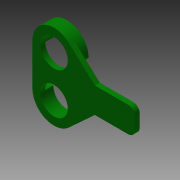
# Autodesk Inventor part: Down Sensor Holder
Saved by Autodesk Inventor 2014 (Build 180170000, 170)
## iProperties
Created: 2016-02-03
Part Number: Down Sensor Holder
Material: Generic
Document SubType Name: Modeling
Designer: Paul
Density: 1 g/cm^3
Appearance: Dark Green
Author: Paul
Autodesk Inventor part; units mm, degrees
ref_plane "YZ Plane" through (0, 0, 0) normal (1, 0, 0) x (0, 1, 0)
ref_plane "XZ Plane" through (0, 0, 0) normal (0, 1, 0) x (-1, 0, 0)
ref_plane "XY Plane" through (0, 0, 0) normal (0, 0, 1) x (1, 0, 0)
sketch "Sketch1" plane through (0, 0, 0) normal (0, 1, 0) x (-1, 0, 0)
  line L0 (-6, 8) -> (15, 8)
  line L1 (15, -8) -> (-6, -8)
  circle A0 centre (40.6, 13.025) radius 8.6
  circle A1 centre (40.6, -13.025) radius 8.6
  line L2 (15, 8) -> (31.4076, 23.048)
  line L3 (54.2, 13.025) -> (54.2, -13.025)
  line L4 (31.4076, -23.048) -> (15, -8)
  line L5 (-10, 0) -> (54.2, 0) construction
  line L6 (32, 21.625) -> (49.2, 21.625) construction
  line L7 (49.2, 21.625) -> (49.2, -21.625) construction
  line L8 (49.2, -21.625) -> (32, -21.625) construction
  line L9 (32, -21.625) -> (32, 21.625) construction
  line L10 (-10, 4) -> (-10, -4)
  arc A2 (-6, 8) -> (-10, 4) centre (-6, 4) ccw
  arc A3 (-10, -4) -> (-6, -8) centre (-6, -4) ccw
  arc A4 (31.4076, -23.048) -> (54.2, -13.025) centre (40.6, -13.025) ccw
  arc A5 (54.2, 13.025) -> (31.4076, 23.048) centre (40.6, 13.025) ccw
  arc A6 (31.4076, 23.048) -> (27, 13.025) centre (40.6, 13.025) ccw construction
  line L11 (32, 13.025) -> (27, 13.025) construction
  line L12 (32, -13.025) -> (27, -13.025) construction
  arc A7 (27, -13.025) -> (31.4076, -23.048) centre (40.6, -13.025) ccw construction
  point P0 (0, 0)
  dimension "d5" = 16
  dimension "d1" = 4
  dimension "d2" = 25
  dimension "d3" = 16
  dimension "d4" = 10
  dimension "d6" = 43.25
  dimension "d10" = 5
  dimension "d22" = 17
  constraints: 26 end point, 12 point on circle, 8 tangent, 6 centre point, 6 parallel, 5 horizontal, 4 coincident, 3 horizontal alignment, 3 vertical, 2 midpoint, 2 perpendicular, 2 point on line, 1 equal radius, 1 symmetric about line, 4 other
  measures "d1" radius of A2
  measures "d2" distance from line of L0.end L10
  measures "d3" distance between parallel lines of L1 L0
  measures "d4" distance from line of L10 point (0, 0)
  measures "d6" distance between parallel lines of L8 L6
  measures "d10" distance between parallel lines of L3 L7
  measures "d22" distance from line of L0.end L9
extrude "Extrusion1" add sketch "Sketch1" along normal blind 3.1
sketch "Sketch2" plane through (0, 3.1, 0) normal (0, 1, 0) x (1, 0, 0)
  line L0 (7.3, -4.8) -> (-7.3, -4.8)
  line L1 (-7.3, -4.8) -> (-7.3, 4.8)
  line L2 (-7.3, 4.8) -> (7.3, 4.8)
  line L3 (7.3, 4.8) -> (7.3, -4.8)
  line L4 (7.3, -4.8) -> (-7.3, 4.8) construction
  line L5 (-7.3, -4.8) -> (7.3, 4.8) construction
  point P0 (0, 0)
  dimension "d14" = 15
  dimension "d15" = 10
  constraints: 12 end point, 2 midpoint, 2 parallel, 1 horizontal, 1 perpendicular
extrude "Extrusion2" add sketch "Sketch2" along normal blind 1.5
fillet "Fillet1" radius 2 4 edges at (7.3, 3.85, 4.8) (-7.3, 3.85, 4.8) (-7.3, 3.85, -4.8) (7.3, 3.85, -4.8)
sketch "Sketch4" plane through (0, 3.1, 0) normal (0, 1, 0) x (1, 0, 0)
  circle A0 centre (-40.6, 13.025) radius 8.6 projected
  circle A1 centre (-40.6, -13.025) radius 8.6 projected
  arc A2 (-31.4076, 23.048) -> (-54.2, 13.025) centre (-40.6, 13.025) ccw projected
  line L0 (10, -4) -> (10, 4) projected
  line L1 (-49.2, 13.025) -> (-54.2, 13.025)
  arc A3 (-27, 13.025) -> (-54.2, 13.025) centre (-40.6, 13.025) ccw
  line L2 (-32, 13.025) -> (-27, 13.025)
  arc A4 (-54.2, -13.025) -> (-31.4076, -23.048) centre (-40.6, -13.025) ccw projected
  line L3 (-15, -8) -> (6, -8) projected
  line L4 (-49.2, -13.025) -> (-54.2, -13.025)
  line L5 (-32, -13.025) -> (-27, -13.025)
  arc A5 (-54.2, -13.025) -> (-27, -13.025) centre (-40.6, -13.025) ccw
  point P0 (0, 0)
  constraints: 8 end point, 8 point on circle, 2 centre point, 2 coincident, 2 collinear, 2 horizontal alignment, 1 parallel, 1 perpendicular
extrude "Extrusion3" add sketch "Sketch4" along normal blind 5 contours A0 L1 A2 A3 L2 | L5 A5 A4 L4 A1
body "Solid1"
